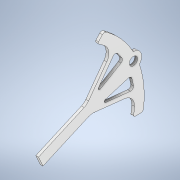
# Autodesk Inventor part: Leg Profile
Saved by Autodesk Inventor 2021 (Build 250183000, 183)
## iProperties
Created: 2021-01-27
Part Number: Leg Profile
Material: UHMW, White
Document SubType Name: Modeling
Designer: M3rob
Density: 0.94 g/cm^3
Appearance: Smooth - White
Author: M3rob
Autodesk Inventor part; units mm, degrees
ref_plane "YZ Plane" through (0, 0, 0) normal (1, 0, 0) x (0, 1, 0)
ref_plane "XZ Plane" through (0, 0, 0) normal (0, 1, 0) x (-1, 0, 0)
ref_plane "XY Plane" through (0, 0, 0) normal (0, 0, 1) x (1, 0, 0)
sketch "Sketch1" plane through (0, 0, 0) normal (0, 1, 0) x (-1, 0, 0)
  line L0 (482.6, -203.2) -> (57.15, -203.2)
  line L1 (-482.6, -203.2) -> (-482.6, 203.2)
  line L2 (-482.6, 203.2) -> (482.6, 203.2)
  line L3 (482.6, 203.2) -> (482.6, -203.2)
  line L4 (57.15, -203.2) -> (57.15, -717.55)
  line L5 (-57.15, -717.55) -> (-57.15, -203.2)
  line L6 (-57.15, -460.375) -> (57.15, -460.375) construction
  line L7 (558.8, -203.2) -> (558.8, 304.8)
  line L8 (-558.8, -203.2) -> (-558.8, 304.8)
  line L9 (0, -460.375) -> (0, 203.2) construction
  line L10 (57.15, -203.2) -> (57.15, 203.2)
  line L11 (-57.15, -203.2) -> (-57.15, 203.2)
  line L12 (-57.15, -50.8) -> (-482.6, -50.8)
  line L13 (57.15, -50.8) -> (482.6, -50.8)
  line L14 (558.8, -203.2) -> (482.6, -203.2)
  line L15 (-558.8, -203.2) -> (-482.6, -203.2)
  line L16 (57.15, -203.2) -> (-482.6, -203.2)
  point P0 (0, 0)
  point P1 (0, -203.2)
  point P2 (-482.6, 0)
  dimension "d1" = 406.4
  dimension "d2" = 920.75
  dimension "d3" = 114.3
  dimension "d4" = 76.2
  dimension "d5" = 508
  dimension "d6" = 152.4
  dimension "d7" = 501.65
  constraints: 34 end point, 10 point on line, 7 perpendicular, 5 midpoint, 4 horizontal, 4 horizontal alignment, 4 vertical, 2 vertical alignment, 1 collinear, 1 other
  measures "d1" distance of L1.start L1.end
  measures "d2" distance from line of L2 L4.end
  measures "d3" distance of L6.start L6.end
  measures "d4" distance between parallel lines of L3 L7
  measures "d5" distance of L8.start L8.end
  measures "d6" distance between parallel lines of L0 L13
  measures "d7" distance of L5.end L8.start
sketch "Sketch2" plane through (0, 0, 0) normal (1, 0, 0) x (0, 1, 0)
  circle A0 centre (101.6, 139.7) radius 101.6 construction
  circle A1 centre (450.85, -654.05) radius 450.85 construction
  line L0 (584.1699, -203.2) -> (0, -203.2) construction
  line L1 (450.85, -654.05) -> (328.0953, -375.062) construction
  circle A2 centre (450.85, -654.05) radius 38.1
  circle A3 centre (101.6, 139.7) radius 82.55 construction
  line L2 (0, 874.2265) -> (0, -722.04) construction
  line L3 (328.0953, -375.062) -> (101.6, 139.7) construction
  line L4 (27.162, 182.7409) -> (212.9696, -239.5491)
  line L5 (305.9656, -198.6309) -> (120.158, 223.6591)
  line L6 (120.158, 223.6591) -> (27.162, 182.7409)
  line L7 (0, -744.1244) -> (0, -722.04) construction
  arc A4 (14.6138, -656.4261) -> (83.1256, -663.6544) centre (127.1252, 81.6881) ccw
  arc A5 (0, -744.1244) -> (22.2106, -747.239) centre (127.1252, 81.6881) ccw construction
  line L8 (766.4539, -331.7414) -> (805.5724, -367.5882)
  line L9 (430.3909, -607.552) -> (471.3091, -700.548) construction
  arc A6 (527.0208, -651.9404) -> (397.8334, -708.7828) centre (450.85, -654.05) ccw construction
  arc A7 (402.924, -713.2914) -> (526.9056, -658.7395) centre (450.85, -654.05) ccw
  arc A8 (533.4061, -648.4236) -> (809.1451, -400.9878) centre (127.1252, 81.6881) ccw
  arc A9 (397.8334, -708.7828) -> (527.0208, -651.9404) centre (127.1252, 81.6881) ccw construction
  arc A10 (533.4061, -648.4236) -> (526.9056, -658.7395) centre (539.5815, -659.5211) ccw
  arc A11 (402.924, -713.2914) -> (390.9266, -711.1145) centre (394.9364, -723.1649) ccw
  line L10 (338.8838, -239.6469) -> (567.4679, -407.2548)
  line L11 (223.9336, -264.4673) -> (220.9696, -291.5291) construction
  line L12 (378.8487, -346.4084) -> (492.4759, -539.6499)
  arc A12 (528.0089, -548.2037) -> (585.3998, -507.7657) centre (127.1252, 81.6881) ccw
  line L13 (584.8292, -467.2295) -> (397.3061, -329.7293)
  line L14 (272.6808, -393.1223) -> (338.3842, -607.4503)
  arc A13 (252.0974, -654.4188) -> (320.6844, -639.4265) centre (127.1252, 81.6881) ccw
  line L15 (222.597, -626.6117) -> (247.914, -395.4618)
  arc A14 (706.3667, -389.4283) -> (747.3244, -334.0334) centre (127.1252, 81.6881) ccw
  arc A15 (180.2773, -663.0577) -> (640.2908, -460.6517) centre (127.1252, 81.6881) ccw construction
  arc A16 (809.1451, -400.9878) -> (805.5724, -367.5882) centre (788.4121, -386.3147) ccw
  arc A17 (0, -722.04) -> (22.2106, -747.239) centre (25.4, -722.04) ccw
  arc A18 (809.1451, -400.9878) -> (821.8545, -382.5085) centre (127.1252, 81.6881) ccw construction
  line L16 (805.5724, -367.5882) -> (821.8545, -382.5085) construction
  arc A19 (22.2106, -747.239) -> (390.9266, -711.1145) centre (127.1252, 81.6881) ccw
  line L17 (0, -722.04) -> (0, -654.05) construction
  line L18 (0, -722.04) -> (0, -668.9811)
  arc A20 (766.4539, -331.7414) -> (747.3244, -334.0334) centre (757.8737, -341.1046) ccw
  arc A21 (14.6138, -656.4261) -> (0, -668.9811) centre (12.7, -668.9811) ccw
  arc A22 (567.4679, -407.2548) -> (706.3667, -389.4283) centre (627.5457, -325.3205) ccw
  arc A23 (83.1256, -663.6544) -> (190.109, -573.2927) centre (89.1129, -562.231) ccw
  arc A24 (305.9656, -198.6309) -> (338.8838, -239.6469) centre (398.9616, -157.7126) ccw
  arc A25 (585.3998, -507.7657) -> (584.8292, -467.2295) centre (569.8097, -487.7131) ccw
  arc A26 (492.4759, -539.6499) -> (528.0089, -548.2037) centre (514.3712, -526.7753) ccw
  arc A27 (397.3061, -329.7293) -> (378.8487, -346.4084) centre (389.7963, -339.9711) ccw
  arc A28 (222.597, -626.6117) -> (252.0974, -654.4188) centre (247.846, -629.3771) ccw
  arc A29 (320.6844, -639.4265) -> (338.3842, -607.4503) centre (314.0997, -614.8948) ccw
  arc A30 (272.6808, -393.1223) -> (247.914, -395.4618) centre (260.5385, -396.8445) ccw
  arc A31 (220.9696, -291.5291) -> (212.9696, -239.5491) centre (119.9736, -280.4674) ccw
  line L19 (212.9696, -239.5491) -> (223.9336, -264.4673) construction
  line L20 (220.9696, -291.5291) -> (190.109, -573.2927)
  point P0 (0, 0)
  point P1 (0, -203.2)
  point P2 (0, 203.2)
  point P3 (0, 203.2)
  point P4 (0, 203.2)
  point P5 (0, 0)
  point P6 (316.9296, -223.5491)
  point P7 (317.9518, -352.0087)
  point P8 (73.66, 203.2)
  point P9 (0, -654.05)
  point P10 (0, -711.2)
  point P11 (755.4457, -321.6539)
  point P12 (347.6183, -293.2961)
  point P13 (505.5773, -561.9309)
  point P14 (611.328, -486.6596)
  point P15 (254.6223, -334.2143)
  point P16 (345.9599, -632.1626)
  point P17 (219.0194, -659.2754)
  dimension "d8" = 203.2
  dimension "d9" = 901.7
  dimension "d10" = 76.2
  dimension "d11" = 63.5
  dimension "d13" = 19.05
  dimension "d15" = 304.8
  dimension "d16" = 101.6
  dimension "d23" = 38.1
  dimension "d24" = 12.7
  dimension "d25" = 12.7
  dimension "d27" = 60
  dimension "d28" = 0
  dimension "d29" = 38.1
  dimension "d30" = 101.6
  dimension "d31" = 25.4
  dimension "d32" = 25.4
  dimension "d33" = 12.7
  dimension "d34" = 12.7
  dimension "d35" = 101.6
  dimension "d36" = 25.4
  dimension "d37" = 12.7
  dimension "d38" = 12.7
  dimension "d39" = 115.9905
  dimension "d40" = 88.9
  constraints: 73 point on circle, 45 tangent, 42 end point, 32 centre point, 25 point on line, 5 coincident, 5 equal radius, 3 symmetric about line, 2 concentric, 2 midpoint, 2 parallel, 2 perpendicular, 2 vertical, 1 collinear, 1 horizontal, 1 horizontal alignment, 4 other
  measures "d8" diameter of A0
  measures "d9" diameter of A1
  measures "d10" diameter of A2
  measures "d11" vertical distance of L3.end point (0, 203.2)
  measures "d13" radial gap between concentric circles of A0 A3
  measures "d15" distance of L1.start L1.end
  measures "d16" distance between parallel lines of L4 L5
  measures "d23" radial gap between concentric circles of A6 A2
  measures "d24" radius of A10
  measures "d25" radius of A11
  measures "d27" angle of L11 L10
  measures "d28" radial gap between concentric circles of A4 A12
  measures "d29" distance between parallel lines of L10 L13
  measures "d30" distance of L9.start L9.end
  measures "d31" radius of A17
  measures "d32" radius of A16
  measures "d33" radius of A20
  measures "d34" radius of A21
  measures "d35" radius of A22
  measures "d36" radius of A25
  measures "d37" radius of A27
  measures "d38" radius of A30
  measures "d39" distance of L14.start L12.start
  measures "d40" radial gap between concentric circles of A19 A15
extrude "Extrusion1" add sketch "Sketch2" along normal mid plane 25.4
body "Solid1"
